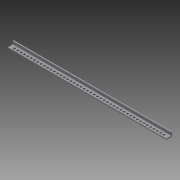
# Autodesk Inventor part: L-Channel Strenght
Saved by Autodesk Inventor 2013 (Build 170138000, 138)
## iProperties
Created: 2013-02-01
Part Number: L-Channel Strenght
Material: Generic
Document SubType Name: Sheet Metal
Designer: actoennies
Density: 1 g/cm^3
Sheet Metal Rule: Default
Flat Pattern Width: 2.51443 cm
Flat Pattern Length: 46.99 cm
Flat Pattern Area: 118.153 cm^2
Sheet Metal Width: 0.990 in
Sheet Metal Length: 18.500 in
Sheet Metal Area: 18.314 in^2
Mass: 32.7238 g
Surface Area: 268.589 cm^2
Volume: 32.7238 cm^3
Author: actoennies
Autodesk Inventor part; units mm, degrees
ref_plane "YZ Plane" through (0, 0, 0) normal (1, 0, 0) x (0, 1, 0)
ref_plane "XZ Plane" through (0, 0, 0) normal (0, 1, 0) x (-1, 0, 0)
ref_plane "XY Plane" through (0, 0, 0) normal (0, 0, 1) x (1, 0, 0)
sketch "Sketch1" plane through (0, 0, 0) normal (0, 1, 0) x (-1, 0, 0)
  line L0 (88.9, -88.9) -> (-381, -88.9)
  circle A0 centre (75.552, -95.25) radius 3.3782
  circle A1 centre (65.7031, -95.25) radius 3.3782
  circle A2 centre (55.8541, -95.25) radius 3.3782
  circle A3 centre (46.0051, -95.25) radius 3.3782
  circle A4 centre (36.1561, -95.25) radius 3.3782
  circle A5 centre (26.3071, -95.25) radius 3.3782
  circle A6 centre (16.4582, -95.25) radius 3.3782
  circle A7 centre (6.6092, -95.25) radius 3.3782
  circle A8 centre (-3.2398, -95.25) radius 3.3782
  circle A9 centre (-13.0888, -95.25) radius 3.3782
  circle A10 centre (-22.9378, -95.25) radius 3.3782
  circle A11 centre (-32.7867, -95.25) radius 3.3782
  circle A12 centre (-42.6357, -95.25) radius 3.3782
  circle A13 centre (-52.4847, -95.25) radius 3.3782
  circle A14 centre (-62.3337, -95.25) radius 3.3782
  circle A15 centre (-72.1827, -95.25) radius 3.3782
  circle A16 centre (-82.0316, -95.25) radius 3.3782
  circle A17 centre (-91.8806, -95.25) radius 3.3782
  circle A18 centre (-101.7296, -95.25) radius 3.3782
  circle A19 centre (-111.5786, -95.25) radius 3.3782
  circle A20 centre (-121.4276, -95.25) radius 3.3782
  circle A21 centre (-131.2765, -95.25) radius 3.3782
  circle A22 centre (-141.1255, -95.25) radius 3.3782
  circle A23 centre (-150.9745, -95.25) radius 3.3782
  circle A24 centre (-160.8235, -95.25) radius 3.3782
  circle A25 centre (-170.6724, -95.25) radius 3.3782
  circle A26 centre (-180.5214, -95.25) radius 3.3782
  circle A27 centre (-190.3704, -95.25) radius 3.3782
  circle A28 centre (-200.2194, -95.25) radius 3.3782
  circle A29 centre (-210.0684, -95.25) radius 3.3782
  circle A30 centre (-219.9173, -95.25) radius 3.3782
  circle A31 centre (-229.7663, -95.25) radius 3.3782
  circle A32 centre (-239.6153, -95.25) radius 3.3782
  circle A33 centre (-249.4643, -95.25) radius 3.3782
  circle A34 centre (-259.3133, -95.25) radius 3.3782
  circle A35 centre (-269.1622, -95.25) radius 3.3782
  circle A36 centre (-279.0112, -95.25) radius 3.3782
  circle A37 centre (-288.8602, -95.25) radius 3.3782
  circle A38 centre (-298.7092, -95.25) radius 3.3782
  circle A39 centre (-308.5582, -95.25) radius 3.3782
  circle A40 centre (-318.4071, -95.25) radius 3.3782
  circle A41 centre (-328.2561, -95.25) radius 3.3782
  circle A42 centre (-338.1051, -95.25) radius 3.3782
  circle A43 centre (-347.9541, -95.25) radius 3.3782
  circle A44 centre (-357.8031, -95.25) radius 3.3782
  circle A45 centre (-367.652, -95.25) radius 3.3782
  line L1 (-381, -88.9) -> (-381, -101.6)
  line L2 (-381, -101.6) -> (88.9, -101.6)
  line L3 (88.9, -88.9) -> (88.9, -101.6)
  point P0 (0, 0)
extrude "Plate1" add sketch "Sketch1" along normal blind 3.175
sketch "Sketch2" plane through (-88.9, 4.445, -102.87) normal (0, 0, -1) x (-1, 0, 0)
  line L0 (-469.9, 0) -> (0, 0)
  line L1 (0, 0) -> (0, 8.255)
  line L2 (0, 8.255) -> (-469.9, 8.255)
  line L3 (-469.9, 8.255) -> (-469.9, 0)
  constraints: 6 end point, 1 horizontal, 1 perpendicular, 1 vertical
edge flange "Flange1" height 12.7 angle 90 thickness 3.175 bend radius 1.27 thickness toward (0, 0, -1) relief straight relief width 3.175 relief depth 1.5875 edges at (146.05, 3.175, -101.6) wall of the first edge with corners at (381, 4.445, -102.87) (-88.9, 4.445, -102.87) (-88.9, 12.7, -102.87) (381, 12.7, -102.87)
bend "Bend1"
corner "Corner1"
equation "\"d1\" = BendReliefWidth"
equation "\"d2\" = BendReliefDepth"
equation "\"d3\" = MinimumRemnant"
equation "\"d4\" = BendRadius"
equation "\"d8\" = CornerReliefSize"
equation "\"d9\" = GapSize"
equation "\"d10\" = JacobiRadiusSize"
equation "\"BendRadius\" = Thickness"
equation "\"BendReliefWidth\" = Thickness"
equation "\"BendReliefDepth\" = 0.5 * Thickness"
equation "\"CornerReliefSize\" = 4 * Thickness"
equation "\"MinimumRemnant\" = 2 * Thickness"
equation "\"TransitionRadius\" = BendRadius"
equation "\"JacobiRadiusSize\" = BendRadius"
equation "\"GapSize\" = Thickness"
equation "\"d0\" = BendRadius"
equation "\"Thickness\" = 3.175"
body "Solid1"
